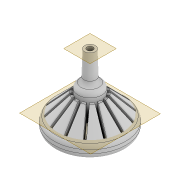
# Autodesk Inventor part: Waterjet_adapter_new_V2
Saved by Autodesk Inventor 2022 (Build 260153000, 153)
## iProperties
Created: 2022-09-02
Part Number: Waterjet_adapter_new_V2
Material: Generic
Document SubType Name: Modeling
Designer: dell
Density: 1 g/cm^3
Appearance: Default
Author: dell
Autodesk Inventor part; units mm, degrees
ref_plane "YZ Plane" through (0, 0, 0) normal (1, 0, 0) x (0, 1, 0)
ref_plane "XZ Plane" through (0, 0, 0) normal (0, 1, 0) x (-1, 0, 0)
ref_plane "XY Plane" through (0, 0, 0) normal (0, 0, 1) x (1, 0, 0)
sketch "Sketch16" plane through (0, 0, 0) normal (0, 1, 0) x (-1, 0, 0)
  circle A0 centre (0, 0) radius 30
  dimension "d82" = 60
  constraints: 1 centre point, 1 coincident
  measures "d82" diameter of A0
extrude "Extrusion11" add sketch "Sketch16" along normal blind 3
sketch "Sketch17" plane through (0, 3, 0) normal (0, 1, 0) x (1, 0, 0)
  circle A0 centre (0, 0) radius 30 projected
  circle A1 centre (0, 0) radius 27
  dimension "d85" = 3
  constraints: 1 centre point
  measures "d85" radial gap between concentric circles of A0 A1
extrude "Extrusion12" add sketch "Sketch17" along normal blind 25
sketch "Sketch18" plane through (0, 3, 0) normal (0, 1, 0) x (1, 0, 0)
  circle A0 centre (0, 0) radius 27 projected
  line L0 (-26.9815, -1) -> (26.9815, -1)
  line L1 (-26.9815, 1) -> (26.9815, 1)
  line L2 (-16.0408, -21.7185) -> (17.6045, 20.4715)
  line L3 (-17.6045, -20.4715) -> (16.0408, 21.7185)
  line L4 (6.9789, -26.0825) -> (-5.029, 26.5275)
  line L5 (5.029, -26.5275) -> (-6.9789, 26.0825)
  line L6 (24.7434, -10.8059) -> (-23.8756, 12.6078)
  line L7 (23.8756, -12.6078) -> (-24.7434, 10.8059)
  line L8 (23.8756, 12.6078) -> (-24.7434, -10.8059)
  line L9 (24.7434, 10.8059) -> (-23.8756, -12.6078)
  line L10 (5.029, 26.5275) -> (-6.9789, -26.0825)
  line L11 (6.9789, 26.0825) -> (-5.029, -26.5275)
  line L12 (-17.6045, 20.4715) -> (16.0408, -21.7185)
  line L13 (-16.0408, 21.7185) -> (17.6045, -20.4715)
  point P0 (-24.7434, -10.8059)
  point P1 (-4.3813, -1)
  point P2 (-3.5135, -2.8019)
  point P3 (-23.8756, -12.6078)
  point P4 (-17.6045, -20.4715)
  point P5 (-6.9789, -26.0825)
  point P6 (-1.9499, -4.0489)
  point P7 (-16.0408, -21.7185)
  point P8 (0, -4.494)
  point P9 (-5.029, -26.5275)
  point P10 (5.029, -26.5275)
  point P11 (1.9499, -4.0489)
  point P12 (6.9789, -26.0825)
  point P13 (3.5135, -2.8019)
  point P14 (17.6045, -20.4715)
  point P15 (4.3813, -1)
  point P16 (24.7434, 10.8059)
  point P17 (4.3813, 1)
  point P18 (3.5135, 2.8019)
  point P19 (6.9789, 26.0825)
  point P20 (1.9499, 4.0489)
  point P21 (0, 4.494)
  point P22 (5.029, 26.5275)
  point P23 (-5.029, 26.5275)
  point P24 (-1.9499, 4.0489)
  point P25 (-6.9789, 26.0825)
  point P26 (-3.5135, 2.8019)
  point P27 (-17.6045, 20.4715)
  point P28 (-4.3813, 1)
  point P29 (-24.7434, 10.8059)
  dimension "d88" = 1
  dimension "d89" = 1
  dimension "d92" = 360
  constraints: 28 end point, 1 horizontal, 48 other
  measures "d88" distance from line of L1 point (0, 0)
  measures "d89" distance from line of point (0, 0) L0
extrude "Extrusion13" add sketch "Sketch18" along normal blind 25 contours L1 L9 A0 | A0 L6 L0 | L8 L2 A0 | A0 L13 L7 | L3 L11 A0 | A0 L4 L12 | L10 L4 A0 | A0 L11 L5 | L5 L13 A0 | A0 L2 L10 | L12 L6 A0 | A0 L9 L3 | L7 L1 A0 | A0 L0 L8
ref_plane "Work Plane7" through (0, 13, 0) normal (0, 1, 0) x (1, 0, 0)
sketch "Sketch20" plane through (0, 13, 0) normal (0, 1, 0) x (1, 0, 0)
  circle A0 centre (0, 0) radius 10
  circle A1 centre (0, 0) radius 2.5
  dimension "d97" = 20
  dimension "d98" = 5
  constraints: 2 centre point, 2 coincident
  measures "d97" diameter of A0
  measures "d98" diameter of A1
extrude "Extrusion14" add sketch "Sketch20" along normal blind 22
chamfer "Chamfer1" distance 18 angle 45 1 edges at (-30, 28, 0)
sketch "Sketch21" plane through (0, 35, 0) normal (0, 1, 0) x (1, 0, 0)
  circle A0 centre (0, 0) radius 5.15
  dimension "d104" = 10.3
  constraints: 1 centre point, 1 coincident
  measures "d104" diameter of A0
ref_plane "Work Plane8" through (0, 60, 0) normal (0, 1, 0) x (1, 0, 0)
sketch "Sketch22" plane through (0, 60, 0) normal (0, 1, 0) x (1, 0, 0)
  circle A0 centre (0, 0) radius 4.5
  dimension "d106" = 9
  constraints: 1 centre point, 1 coincident
  measures "d106" diameter of A0
loft "Loft3" add profiles "Sketch21", "Sketch22"
sketch "Sketch23" plane through (0, 60, 0) normal (0, 1, 0) x (1, 0, 0)
  circle A0 centre (0, 0) radius 2.5
  dimension "d111" = 5
  constraints: 1 centre point, 1 coincident
  measures "d111" diameter of A0
extrude "Extrusion15" cut sketch "Sketch23" against normal blind 35
fillet "Fillet3" radius 5 2 edges at (-5.15, 35, 0) (-10, 35, 0)
fillet "Fillet4" radius 5 2 edges at (30, 0, 0) (-30, 10, 0)
fillet "Fillet5" radius 3 1 edges at (-2.5, 13, 0)
body "Solid2"
